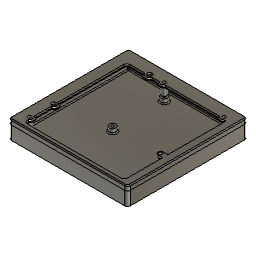
Lightroom-Macropad-Case (Autodesk Fusion 360 design; units mm, degrees)
Autodesk Fusion 360 part; units mm, degrees
(part 1 of 2)
sketch "BoardSVG" plane through (0, 0, 0) normal (0, 0, 1) x (1, 0, 0)
  ellipse E0 centre (-23.8658, -18.9665) end of major axis (-23.0959, -18.9665) minor radius 0.7699
  circle A0 centre (-23.8661, -18.9665) radius 0.5052
  ellipse E1 centre (-8.2045, -18.9665) end of major axis (-7.4346, -18.9665) minor radius 0.7699
  circle A1 centre (-8.2047, -18.9665) radius 0.5052
  ellipse E2 centre (-23.8658, -11.2672) end of major axis (-23.0959, -11.2672) minor radius 0.7699
  circle A2 centre (-23.8661, -11.2672) radius 0.5052
  ellipse E3 centre (-8.2045, -11.2672) end of major axis (-7.4346, -11.2672) minor radius 0.7699
  circle A3 centre (-8.2047, -11.2672) radius 0.5052
  ellipse E4 centre (-23.8658, -4.851) end of major axis (-23.0959, -4.851) minor radius 0.7699
  circle A4 centre (-23.8661, -4.851) radius 0.5052
  ellipse E5 centre (-8.2045, -4.851) end of major axis (-7.4346, -4.851) minor radius 0.7699
  circle A5 centre (-8.2047, -4.851) radius 0.5052
  ellipse E6 centre (-23.8658, 1.5651) end of major axis (-23.0959, 1.5651) minor radius 0.7699
  circle A6 centre (-23.8661, 1.5651) radius 0.5052
  ellipse E7 centre (-8.2045, 1.5651) end of major axis (-7.4346, 1.5651) minor radius 0.7699
  circle A7 centre (-8.2047, 1.5651) radius 0.5052
  ellipse E8 centre (66.4399, -35.8623) end of major axis (67.2482, -35.8623) minor radius 0.8083
  circle A8 centre (66.44, -35.8624) radius 0.4042
  ellipse E9 centre (74.7254, -35.8623) end of major axis (75.5338, -35.8623) minor radius 0.8083
  circle A9 centre (74.7254, -35.8624) radius 0.4042
  ellipse E10 centre (66.4399, -40.5676) end of major axis (67.2482, -40.5676) minor radius 0.8083
  circle A10 centre (66.44, -40.5676) radius 0.4042
  ellipse E11 centre (74.7254, -40.5676) end of major axis (75.5338, -40.5676) minor radius 0.8083
  circle A11 centre (74.7254, -40.5676) radius 0.4042
  ellipse E12 centre (66.4399, -45.2727) end of major axis (67.2482, -45.2727) minor radius 0.8083
  circle A12 centre (66.44, -45.2727) radius 0.4042
  ellipse E13 centre (74.7254, -45.2727) end of major axis (75.5338, -45.2727) minor radius 0.8083
  circle A13 centre (74.7254, -45.2727) radius 0.4042
  ellipse E14 centre (13.8275, 10.5477) end of major axis (14.6358, 10.5477) minor radius 0.8083
  circle A14 centre (13.8276, 10.5477) radius 0.4042
  ellipse E15 centre (22.113, 10.5477) end of major axis (22.9214, 10.5477) minor radius 0.8083
  circle A15 centre (22.113, 10.5477) radius 0.4042
  ellipse E16 centre (13.8275, 1.5651) end of major axis (14.6358, 1.5651) minor radius 0.8083
  circle A16 centre (13.8276, 1.5651) radius 0.4042
  ellipse E17 centre (22.113, 1.5651) end of major axis (22.9214, 1.5651) minor radius 0.8083
  circle A17 centre (22.113, 1.5651) radius 0.4042
  ellipse E18 centre (13.8275, -2.9262) end of major axis (14.6358, -2.9262) minor radius 0.8083
  circle A18 centre (13.8276, -2.9262) radius 0.4042
  ellipse E19 centre (22.113, -2.9262) end of major axis (22.9214, -2.9262) minor radius 0.8083
  circle A19 centre (22.113, -2.9262) radius 0.4042
  ellipse E20 centre (27.943, -45.2727) end of major axis (28.7513, -45.2727) minor radius 0.8083
  circle A20 centre (27.9431, -45.2727) radius 0.4042
  ellipse E21 centre (36.2286, -45.2727) end of major axis (37.0369, -45.2727) minor radius 0.8083
  circle A21 centre (36.2285, -45.2727) radius 0.4042
  ellipse E22 centre (27.943, -40.5674) end of major axis (28.7513, -40.5674) minor radius 0.8083
  circle A22 centre (27.9431, -40.5676) radius 0.4042
  ellipse E23 centre (36.2286, -40.5674) end of major axis (37.0369, -40.5674) minor radius 0.8083
  circle A23 centre (36.2285, -40.5676) radius 0.4042
  ellipse E24 centre (27.943, -31.1572) end of major axis (28.7513, -31.1572) minor radius 0.8083
  circle A24 centre (27.9431, -31.1572) radius 0.4042
  ellipse E25 centre (36.2286, -31.1572) end of major axis (37.0369, -31.1572) minor radius 0.8083
  circle A25 centre (36.2285, -31.1572) radius 0.4042
  ellipse E26 centre (27.943, -35.8623) end of major axis (28.7513, -35.8623) minor radius 0.8083
  circle A26 centre (27.9431, -35.8624) radius 0.4042
  ellipse E27 centre (36.2286, -35.8623) end of major axis (37.0369, -35.8623) minor radius 0.8083
  circle A27 centre (36.2285, -35.8624) radius 0.4042
  ellipse E28 centre (13.8275, -55.1107) end of major axis (14.6358, -55.1107) minor radius 0.8083
  circle A28 centre (13.8276, -55.1108) radius 0.4042
  ellipse E29 centre (22.113, -55.1107) end of major axis (22.9214, -55.1107) minor radius 0.8083
  circle A29 centre (22.113, -55.1108) radius 0.4042
  ellipse E30 centre (13.8275, -59.8161) end of major axis (14.6358, -59.8161) minor radius 0.8083
  circle A30 centre (13.8276, -59.816) radius 0.4042
  ellipse E31 centre (22.113, -59.8161) end of major axis (22.9214, -59.8161) minor radius 0.8083
  circle A31 centre (22.113, -59.816) radius 0.4042
  ellipse E32 centre (13.8275, -64.5212) end of major axis (14.6358, -64.5212) minor radius 0.8083
  circle A32 centre (13.8276, -64.5212) radius 0.4042
  ellipse E33 centre (22.113, -64.5212) end of major axis (22.9214, -64.5212) minor radius 0.8083
  circle A33 centre (22.113, -64.5212) radius 0.4042
  ellipse E34 centre (66.4399, -31.1572) end of major axis (67.2482, -31.1572) minor radius 0.8083
  circle A34 centre (66.44, -31.1572) radius 0.4042
  ellipse E35 centre (74.7254, -31.1572) end of major axis (75.5338, -31.1572) minor radius 0.8083
  circle A35 centre (74.7254, -31.1572) radius 0.4042
  ellipse E36 centre (13.8275, 6.0564) end of major axis (14.6358, 6.0564) minor radius 0.8083
  circle A36 centre (13.8276, 6.0564) radius 0.4042
  ellipse E37 centre (22.113, 6.0564) end of major axis (22.9214, 6.0564) minor radius 0.8083
  circle A37 centre (22.113, 6.0564) radius 0.4042
  ellipse E38 centre (13.8275, -50.4056) end of major axis (14.6358, -50.4056) minor radius 0.8083
  circle A38 centre (13.8276, -50.4056) radius 0.4042
  ellipse E39 centre (22.113, -50.4056) end of major axis (22.9214, -50.4056) minor radius 0.8083
  circle A39 centre (22.113, -50.4056) radius 0.4042
  ellipse E40 centre (-6.2799, -53.6137) end of major axis (-5.51, -53.6137) minor radius 0.7699
  circle A40 centre (-6.2797, -53.6137) radius 0.5052
  ellipse E41 centre (-21.941, -53.6137) end of major axis (-21.1711, -53.6137) minor radius 0.7699
  circle A41 centre (-21.9411, -53.6137) radius 0.5052
  ellipse E42 centre (17.9703, 16.1909) end of major axis (18.7402, 16.1909) minor radius 0.7699
  circle A42 centre (17.9703, 16.1909) radius 0.5052
  ellipse E43 centre (17.9703, 31.8522) end of major axis (18.7402, 31.8522) minor radius 0.7699
  circle A43 centre (17.9703, 31.8523) radius 0.5052
  ellipse E44 centre (-21.1682, -36.9317) end of major axis (-20.4609, -36.9317) minor radius 0.7073
  circle A44 centre (-21.1682, -36.9317) radius 0.4547
  ellipse E45 centre (-21.1682, -39.4982) end of major axis (-20.4609, -39.4982) minor radius 0.7073
  circle A45 centre (-21.1682, -39.4982) radius 0.4547
  ellipse E46 centre (3.2131, 40.7036) end of major axis (3.9204, 40.7036) minor radius 0.7073
  circle A46 centre (3.2131, 40.7036) radius 0.4547
  ellipse E47 centre (3.2131, 38.1372) end of major axis (3.9204, 38.1372) minor radius 0.7073
  circle A47 centre (3.2131, 38.1372) radius 0.4547
  ellipse E48 centre (17.9703, -15.1168) end of major axis (21.5067, -15.1168) minor radius 3.5365
  circle A48 centre (17.9703, -15.1168) radius 1.7965
  ellipse E49 centre (28.2361, 25.9465) end of major axis (29.4486, 25.9465) minor radius 1.2125
  circle A49 centre (28.2361, 25.9465) radius 0.8083
  ellipse E50 centre (34.6522, 28.5129) end of major axis (35.8647, 28.5129) minor radius 1.2125
  circle A50 centre (34.6522, 28.5129) radius 0.8083
  ellipse E51 centre (47.4845, 25.9465) end of major axis (48.697, 25.9465) minor radius 1.2125
  circle A51 centre (47.4845, 25.9465) radius 0.8083
  ellipse E52 centre (53.9007, 28.5129) end of major axis (55.1132, 28.5129) minor radius 1.2125
  circle A52 centre (53.9007, 28.5129) radius 0.8083
  ellipse E53 centre (-10.2608, -35.6485) end of major axis (-9.0483, -35.6485) minor radius 1.2125
  circle A53 centre (-10.2608, -35.6485) radius 0.8083
  ellipse E54 centre (-3.8446, -33.0821) end of major axis (-2.6321, -33.0821) minor radius 1.2125
  circle A54 centre (-3.8446, -33.0821) radius 0.8083
  ellipse E55 centre (8.9877, -35.6485) end of major axis (10.2002, -35.6485) minor radius 1.2125
  circle A55 centre (8.9877, -35.6485) radius 0.8083
  ellipse E56 centre (15.4038, -33.0821) end of major axis (16.6163, -33.0821) minor radius 1.2125
  circle A56 centre (15.4038, -33.0821) radius 0.8083
  ellipse E57 centre (66.733, -12.5504) end of major axis (67.9455, -12.5504) minor radius 1.2125
  circle A57 centre (66.733, -12.5504) radius 0.8083
  ellipse E58 centre (73.1491, -9.9839) end of major axis (74.3616, -9.9839) minor radius 1.2125
  circle A58 centre (73.1491, -9.9839) radius 0.8083
  ellipse E59 centre (66.733, 25.9465) end of major axis (67.9455, 25.9465) minor radius 1.2125
  circle A59 centre (66.733, 25.9465) radius 0.8083
  ellipse E60 centre (73.1491, 28.5129) end of major axis (74.3616, 28.5129) minor radius 1.2125
  circle A60 centre (73.1491, 28.5129) radius 0.8083
  ellipse E61 centre (47.4845, -54.8969) end of major axis (48.697, -54.8969) minor radius 1.2125
  circle A61 centre (47.4845, -54.8969) radius 0.8083
  ellipse E62 centre (53.9007, -52.3305) end of major axis (55.1132, -52.3305) minor radius 1.2125
  circle A62 centre (53.9007, -52.3305) radius 0.8083
  ellipse E63 centre (0.0051, -54.8969) end of major axis (1.2175, -54.8969) minor radius 1.2125
  circle A63 centre (0.0051, -54.8969) radius 0.8083
  ellipse E64 centre (6.4212, -52.3305) end of major axis (7.6337, -52.3305) minor radius 1.2125
  circle A64 centre (6.4212, -52.3305) radius 0.8083
  ellipse E65 centre (28.2361, -54.8969) end of major axis (29.4486, -54.8969) minor radius 1.2125
  circle A65 centre (28.2361, -54.8969) radius 0.8083
  ellipse E66 centre (34.6522, -52.3305) end of major axis (35.8647, -52.3305) minor radius 1.2125
  circle A66 centre (34.6522, -52.3305) radius 0.8083
  ellipse E67 centre (66.733, 6.6981) end of major axis (67.9455, 6.6981) minor radius 1.2125
  circle A67 centre (66.733, 6.6981) radius 0.8083
  ellipse E68 centre (73.1491, 9.2645) end of major axis (74.3616, 9.2645) minor radius 1.2125
  circle A68 centre (73.1491, 9.2645) radius 0.8083
  ellipse E69 centre (47.4845, -12.5504) end of major axis (48.697, -12.5504) minor radius 1.2125
  circle A69 centre (47.4845, -12.5504) radius 0.8083
  ellipse E70 centre (53.9007, -9.9839) end of major axis (55.1132, -9.9839) minor radius 1.2125
  circle A70 centre (53.9007, -9.9839) radius 0.8083
  ellipse E71 centre (28.2361, 6.6981) end of major axis (29.4486, 6.6981) minor radius 1.2125
  circle A71 centre (28.2361, 6.6981) radius 0.8083
  ellipse E72 centre (34.6522, 9.2645) end of major axis (35.8647, 9.2645) minor radius 1.2125
  circle A72 centre (34.6522, 9.2645) radius 0.8083
  ellipse E73 centre (66.733, -54.8969) end of major axis (67.9455, -54.8969) minor radius 1.2125
  circle A73 centre (66.733, -54.8969) radius 0.8083
  ellipse E74 centre (73.1491, -52.3305) end of major axis (74.3616, -52.3305) minor radius 1.2125
  circle A74 centre (73.1491, -52.3305) radius 0.8083
  ellipse E75 centre (28.2361, -12.5504) end of major axis (29.4486, -12.5504) minor radius 1.2125
  circle A75 centre (28.2361, -12.5504) radius 0.8083
  ellipse E76 centre (34.6522, -9.9839) end of major axis (35.8647, -9.9839) minor radius 1.2125
  circle A76 centre (34.6522, -9.9839) radius 0.8083
  ellipse E77 centre (47.4845, 6.6981) end of major axis (48.697, 6.6981) minor radius 1.2125
  circle A77 centre (47.4845, 6.6981) radius 0.8083
  ellipse E78 centre (53.9007, 9.2645) end of major axis (55.1132, 9.2645) minor radius 1.2125
  circle A78 centre (53.9007, 9.2645) radius 0.8083
  ellipse E79 centre (47.4845, -35.6485) end of major axis (48.697, -35.6485) minor radius 1.2125
  circle A79 centre (47.4845, -35.6485) radius 0.8083
  ellipse E80 centre (53.9007, -33.0821) end of major axis (55.1132, -33.0821) minor radius 1.2125
  circle A80 centre (53.9007, -33.0821) radius 0.8083
  ellipse E81 centre (17.9703, 38.7788) end of major axis (21.5067, 38.7788) minor radius 3.5365
  circle A81 centre (17.9703, 38.7788) radius 1.7965
  ellipse E82 centre (80.2069, 38.7788) end of major axis (83.7433, 38.7788) minor radius 3.5365
  circle A82 centre (80.2069, 38.7788) radius 1.7965
  ellipse E83 centre (-21.1682, -62.5963) end of major axis (-17.6318, -62.5963) minor radius 3.5365
  circle A83 centre (-21.1682, -62.5963) radius 1.7965
  ellipse E84 centre (80.2069, -27.3075) end of major axis (83.7433, -27.3075) minor radius 3.5365
  circle A84 centre (80.2069, -27.3075) radius 1.7965
  line L0 (-24.5046, 40.1903) -> (-22.9647, 40.1903)
  line L1 (-22.9647, 40.1903) -> (-22.9647, 38.6505)
  line L2 (-22.9647, 38.6505) -> (-24.5046, 38.6505)
  line L3 (-24.5046, 38.6505) -> (-24.5046, 40.1903)
  circle A85 centre (-23.7347, 39.4204) radius 0.462
  ellipse E85 centre (-23.7347, 36.8539) end of major axis (-22.9647, 36.8539) minor radius 0.7699
  circle A86 centre (-23.7347, 36.8539) radius 0.462
  ellipse E86 centre (-23.7347, 31.721) end of major axis (-22.9647, 31.721) minor radius 0.7699
  circle A87 centre (-23.7347, 31.721) radius 0.462
  ellipse E87 centre (-23.7347, 29.1546) end of major axis (-22.9647, 29.1546) minor radius 0.7699
  circle A88 centre (-23.7347, 29.1546) radius 0.462
  ellipse E88 centre (-23.7347, 26.5881) end of major axis (-22.9647, 26.5881) minor radius 0.7699
  circle A89 centre (-23.7347, 26.5881) radius 0.462
  ellipse E89 centre (-23.7347, 24.0216) end of major axis (-22.9647, 24.0216) minor radius 0.7699
  circle A90 centre (-23.7347, 24.0216) radius 0.462
  ellipse E90 centre (-23.7347, 21.4552) end of major axis (-22.9647, 21.4552) minor radius 0.7699
  circle A91 centre (-23.7347, 21.4552) radius 0.462
  ellipse E91 centre (-23.7347, 18.8887) end of major axis (-22.9647, 18.8887) minor radius 0.7699
  circle A92 centre (-23.7347, 18.8887) radius 0.462
  ellipse E92 centre (-23.7347, 16.3223) end of major axis (-22.9647, 16.3223) minor radius 0.7699
  circle A93 centre (-23.7347, 16.3223) radius 0.462
  ellipse E93 centre (-23.7347, 13.7558) end of major axis (-22.9647, 13.7558) minor radius 0.7699
  circle A94 centre (-23.7347, 13.7558) radius 0.462
  ellipse E94 centre (-23.7347, 11.1894) end of major axis (-22.9647, 11.1894) minor radius 0.7699
  circle A95 centre (-23.7347, 11.1894) radius 0.462
  ellipse E95 centre (-8.3359, 11.1894) end of major axis (-7.566, 11.1894) minor radius 0.7699
  circle A96 centre (-8.3359, 11.1894) radius 0.462
  ellipse E96 centre (-8.3359, 13.7558) end of major axis (-7.566, 13.7558) minor radius 0.7699
  circle A97 centre (-8.3359, 13.7558) radius 0.462
  ellipse E97 centre (-8.3359, 16.3223) end of major axis (-7.566, 16.3223) minor radius 0.7699
  circle A98 centre (-8.3359, 16.3223) radius 0.462
  ellipse E98 centre (-8.3359, 18.8887) end of major axis (-7.566, 18.8887) minor radius 0.7699
  circle A99 centre (-8.3359, 18.8887) radius 0.462
  ellipse E99 centre (-8.3359, 21.4552) end of major axis (-7.566, 21.4552) minor radius 0.7699
  circle A100 centre (-8.3359, 21.4552) radius 0.462
  ellipse E100 centre (-8.3359, 24.0216) end of major axis (-7.566, 24.0216) minor radius 0.7699
  circle A101 centre (-8.3359, 24.0216) radius 0.462
  ellipse E101 centre (-8.3359, 26.5881) end of major axis (-7.566, 26.5881) minor radius 0.7699
  circle A102 centre (-8.3359, 26.5881) radius 0.462
  ellipse E102 centre (-8.3359, 29.1546) end of major axis (-7.566, 29.1546) minor radius 0.7699
  circle A103 centre (-8.3359, 29.1546) radius 0.462
  ellipse E103 centre (-8.3359, 31.721) end of major axis (-7.566, 31.721) minor radius 0.7699
  circle A104 centre (-8.3359, 31.721) radius 0.462
  ellipse E104 centre (-8.3359, 34.2875) end of major axis (-7.566, 34.2875) minor radius 0.7699
  circle A105 centre (-8.3359, 34.2875) radius 0.462
  ellipse E105 centre (-8.3359, 36.8539) end of major axis (-7.566, 36.8539) minor radius 0.7699
  circle A106 centre (-8.3359, 36.8539) radius 0.462
  ellipse E106 centre (-8.3359, 39.4204) end of major axis (-7.566, 39.4204) minor radius 0.7699
  circle A107 centre (-8.3359, 39.4204) radius 0.462
  ellipse E107 centre (-23.7347, 34.2875) end of major axis (-22.9647, 34.2875) minor radius 0.7699
  circle A108 centre (-23.7347, 34.2875) radius 0.462
  ellipse E108 centre (-1.9198, -23.9578) end of major axis (-0.6568, -23.9578) minor radius 1.263
  circle A109 centre (-1.9198, -23.9578) radius 0.8083
  ellipse E109 centre (3.2131, -23.958) end of major axis (4.4761, -23.958) minor radius 1.263
  circle A110 centre (3.2131, -23.958) radius 0.8083
  ellipse E110 centre (8.346, -23.9578) end of major axis (9.6091, -23.9578) minor radius 1.263
  circle A111 centre (8.346, -23.9578) radius 0.8083
  ellipse E111 centre (0.6467, -6.2757) end of major axis (1.9097, -6.2757) minor radius 1.263
  circle A112 centre (0.6467, -6.2757) radius 0.8083
  ellipse E112 centre (5.7796, -6.2757) end of major axis (7.0426, -6.2757) minor radius 1.263
  circle A113 centre (5.7796, -6.2757) radius 0.8083
  arc A114 (-5.8806, -13.197) -> (-2.6474, -13.197) centre (-4.264, -13.2073) cw
  line L4 (-2.6474, -13.197) -> (-2.6474, -13.5002)
  arc A115 (-2.6474, -13.5002) -> (-5.8806, -13.5002) centre (-4.264, -13.4899) cw
  line L5 (-5.8806, -13.5002) -> (-5.8806, -13.197)
  arc A116 (-3.0514, -13.3991) -> (-5.4765, -13.3991) centre (-4.2639, -13.3991) cw
  line L6 (-5.4765, -13.3991) -> (-5.4765, -13.298)
  arc A117 (-5.4765, -13.298) -> (-3.0514, -13.298) centre (-4.2639, -13.298) cw
  line L7 (-3.0514, -13.298) -> (-3.0514, -13.3991)
  arc A118 (9.0736, -13.197) -> (12.3069, -13.197) centre (10.6903, -13.2073) cw
  line L8 (12.3069, -13.197) -> (12.3069, -13.5002)
  arc A119 (12.3069, -13.5002) -> (9.0736, -13.5002) centre (10.6903, -13.4899) cw
  line L9 (9.0736, -13.5002) -> (9.0736, -13.197)
  arc A120 (11.9027, -13.3991) -> (9.4776, -13.3991) centre (10.6902, -13.3991) cw
  line L10 (9.4776, -13.3991) -> (9.4776, -13.298)
  arc A121 (9.4776, -13.298) -> (11.9027, -13.298) centre (10.6902, -13.298) cw
  line L11 (11.9027, -13.298) -> (11.9027, -13.3991)
  ellipse E113 centre (-1.9198, 3.6316) end of major axis (-0.6568, 3.6316) minor radius 1.263
  circle A122 centre (-1.9198, 3.6316) radius 0.8083
  ellipse E114 centre (3.2131, 3.6314) end of major axis (4.4761, 3.6314) minor radius 1.263
  circle A123 centre (3.2131, 3.6314) radius 0.8083
  ellipse E115 centre (8.346, 3.6316) end of major axis (9.6091, 3.6316) minor radius 1.263
  circle A124 centre (8.346, 3.6316) radius 0.8083
  ellipse E116 centre (0.6467, 21.3138) end of major axis (1.9097, 21.3138) minor radius 1.263
  circle A125 centre (0.6467, 21.3138) radius 0.8083
  ellipse E117 centre (5.7796, 21.3138) end of major axis (7.0426, 21.3138) minor radius 1.263
  circle A126 centre (5.7796, 21.3138) radius 0.8083
  arc A127 (-5.8806, 14.3924) -> (-2.6474, 14.3924) centre (-4.264, 14.3821) cw
  line L12 (-2.6474, 14.3924) -> (-2.6474, 14.0893)
  arc A128 (-2.6474, 14.0893) -> (-5.8806, 14.0893) centre (-4.264, 14.0996) cw
  line L13 (-5.8806, 14.0893) -> (-5.8806, 14.3924)
  arc A129 (-3.0514, 14.1903) -> (-5.4765, 14.1903) centre (-4.2639, 14.1903) cw
  line L14 (-5.4765, 14.1903) -> (-5.4765, 14.2914)
  arc A130 (-5.4765, 14.2914) -> (-3.0514, 14.2914) centre (-4.2639, 14.2914) cw
  line L15 (-3.0514, 14.2914) -> (-3.0514, 14.1903)
  arc A131 (9.0736, 14.3924) -> (12.3069, 14.3924) centre (10.6903, 14.3821) cw
  line L16 (12.3069, 14.3924) -> (12.3069, 14.0893)
  arc A132 (12.3069, 14.0893) -> (9.0736, 14.0893) centre (10.6903, 14.0996) cw
  line L17 (9.0736, 14.0893) -> (9.0736, 14.3924)
  arc A133 (11.9027, 14.1903) -> (9.4776, 14.1903) centre (10.6902, 14.1903) cw
  line L18 (9.4776, 14.1903) -> (9.4776, 14.2914)
  arc A134 (9.4776, 14.2914) -> (11.9027, 14.2914) centre (10.6902, 14.2914) cw
  line L19 (11.9027, 14.2914) -> (11.9027, 14.1903)
  circle A135 centre (27.8396, 3.4733) radius 0.3082
  circle A136 centre (27.8396, 3.4733) radius 0.1541
  circle A137 centre (47.4576, -38.3589) radius 0.3082
  circle A138 centre (47.4576, -38.3589) radius 0.1541
  circle A139 centre (28.5045, 24.247) radius 0.3082
  circle A140 centre (28.5045, 24.247) radius 0.1541
  circle A141 centre (22.8011, 8.6693) radius 0.3082
  circle A142 centre (22.8011, 8.6693) radius 0.1541
  circle A143 centre (26.271, 4.7039) radius 0.3082
  circle A144 centre (26.271, 4.7039) radius 0.1541
  circle A145 centre (-7.4264, -0.6107) radius 0.3082
  circle A146 centre (-7.4264, -0.6107) radius 0.1541
  circle A147 centre (-15.7933, 7.1659) radius 0.3082
  circle A148 centre (-15.7933, 7.1659) radius 0.1541
  circle A149 centre (-3.6532, 5.7888) radius 0.3082
  circle A150 centre (-3.6532, 5.7888) radius 0.1541
  circle A151 centre (22.6764, -27.2341) radius 0.3082
  circle A152 centre (22.6764, -27.2341) radius 0.1541
  line L20 (-22.3231, 46.2215) -> (82.9017, 46.2215)
  line L21 (82.9017, -69.2691) -> (-22.3231, -69.2691)
  line L22 (-27.4561, -64.1362) -> (-27.4561, 41.0886)
  line L23 (88.0346, 41.0886) -> (88.0346, -64.1362)
  arc A153 (82.9017, 46.2215) -> (88.0346, 41.0886) centre (82.9017, 41.0886) cw
  arc A154 (88.0346, -64.1362) -> (82.9017, -69.2691) centre (82.9017, -64.1362) cw
  arc A155 (-22.3231, -69.2691) -> (-27.4561, -64.1362) centre (-22.3231, -64.1362) cw
  arc A156 (-27.4561, 41.0886) -> (-22.3231, 46.2215) centre (-22.3231, 41.0886) cw
  point P0 (-23.0959, -18.9665)
  point P1 (-23.3609, -18.9665)
  point P2 (-7.4346, -18.9665)
  point P3 (-7.6995, -18.9665)
  point P4 (-23.0959, -11.2672)
  point P5 (-23.3609, -11.2672)
  point P6 (-7.4346, -11.2672)
  point P7 (-7.6995, -11.2672)
  point P8 (-23.0959, -4.851)
  point P9 (-23.3609, -4.851)
  point P10 (-7.4346, -4.851)
  point P11 (-7.6995, -4.851)
  point P12 (-23.0959, 1.5651)
  point P13 (-23.3609, 1.5651)
  point P14 (-7.4346, 1.5651)
  point P15 (-7.6995, 1.5651)
  point P16 (67.2482, -35.8623)
  point P17 (66.8441, -35.8624)
  point P18 (75.5338, -35.8623)
  point P19 (75.1295, -35.8624)
  point P20 (67.2482, -40.5676)
  point P21 (66.8441, -40.5676)
  point P22 (75.5338, -40.5676)
  point P23 (75.1295, -40.5676)
  point P24 (67.2482, -45.2727)
  point P25 (66.8441, -45.2727)
  point P26 (75.5338, -45.2727)
  point P27 (75.1295, -45.2727)
  point P28 (14.6358, 10.5477)
  point P29 (14.2317, 10.5477)
  point P30 (22.9214, 10.5477)
  point P31 (22.5171, 10.5477)
  point P32 (14.6358, 1.5651)
  point P33 (14.2317, 1.5651)
  point P34 (22.9214, 1.5651)
  point P35 (22.5171, 1.5651)
  point P36 (14.6358, -2.9262)
  point P37 (14.2317, -2.9262)
  point P38 (22.9214, -2.9262)
  point P39 (22.5171, -2.9262)
  point P40 (28.7513, -45.2727)
  point P41 (28.3472, -45.2727)
  point P42 (37.0369, -45.2727)
  point P43 (36.6326, -45.2727)
  point P44 (28.7513, -40.5674)
  point P45 (28.3472, -40.5676)
  point P46 (37.0369, -40.5674)
  point P47 (36.6326, -40.5676)
  point P48 (28.7513, -31.1572)
  point P49 (28.3472, -31.1572)
  point P50 (37.0369, -31.1572)
  point P51 (36.6326, -31.1572)
  point P52 (28.7513, -35.8623)
  point P53 (28.3472, -35.8624)
  point P54 (37.0369, -35.8623)
  point P55 (36.6326, -35.8624)
  point P56 (14.6358, -55.1107)
  point P57 (14.2317, -55.1108)
  point P58 (22.9214, -55.1107)
  point P59 (22.5171, -55.1108)
  point P60 (14.6358, -59.8161)
  point P61 (14.2317, -59.816)
  point P62 (22.9214, -59.8161)
  point P63 (22.5171, -59.816)
  point P64 (14.6358, -64.5212)
  point P65 (14.2317, -64.5212)
  point P66 (22.9214, -64.5212)
  point P67 (22.5171, -64.5212)
  point P68 (67.2482, -31.1572)
  point P69 (66.8441, -31.1572)
  point P70 (75.5338, -31.1572)
  point P71 (75.1295, -31.1572)
  point P72 (14.6358, 6.0564)
  point P73 (14.2317, 6.0564)
  point P74 (22.9214, 6.0564)
  point P75 (22.5171, 6.0564)
  point P76 (14.6358, -50.4056)
  point P77 (14.2317, -50.4056)
  point P78 (22.9214, -50.4056)
  point P79 (22.5171, -50.4056)
  point P80 (-5.51, -53.6137)
  point P81 (-5.7745, -53.6137)
  point P82 (-21.1711, -53.6137)
  point P83 (-21.4359, -53.6137)
  point P84 (18.7402, 16.1909)
  point P85 (18.4755, 16.1909)
  point P86 (18.7402, 31.8522)
  point P87 (18.4755, 31.8523)
  point P88 (-20.4609, -36.9317)
  point P89 (-20.7135, -36.9317)
  point P90 (-20.4609, -39.4982)
  point P91 (-20.7135, -39.4982)
  point P92 (3.9204, 40.7036)
  point P93 (3.6678, 40.7036)
  point P94 (3.9204, 38.1372)
  point P95 (3.6678, 38.1372)
  point P96 (21.5067, -15.1168)
  point P97 (19.7668, -15.1168)
  point P98 (29.4486, 25.9465)
  point P99 (29.0444, 25.9465)
  point P100 (35.8647, 28.5129)
  point P101 (35.4606, 28.5129)
  point P102 (48.697, 25.9465)
  point P103 (48.2929, 25.9465)
  point P104 (55.1132, 28.5129)
  point P105 (54.709, 28.5129)
  point P106 (-9.0483, -35.6485)
  point P107 (-9.4524, -35.6485)
  point P108 (-2.6321, -33.0821)
  point P109 (-3.0363, -33.0821)
  point P110 (10.2002, -35.6485)
  point P111 (9.796, -35.6485)
  point P112 (16.6163, -33.0821)
  point P113 (16.2121, -33.0821)
  point P114 (67.9455, -12.5504)
  point P115 (67.5413, -12.5504)
  point P116 (74.3616, -9.9839)
  point P117 (73.9574, -9.9839)
  point P118 (67.9455, 25.9465)
  point P119 (67.5413, 25.9465)
  point P120 (74.3616, 28.5129)
  point P121 (73.9574, 28.5129)
  point P122 (48.697, -54.8969)
  point P123 (48.2929, -54.8969)
  point P124 (55.1132, -52.3305)
  point P125 (54.709, -52.3305)
  point P126 (1.2175, -54.8969)
  point P127 (0.8134, -54.8969)
  point P128 (7.6337, -52.3305)
  point P129 (7.2295, -52.3305)
  point P130 (29.4486, -54.8969)
  point P131 (29.0444, -54.8969)
  point P132 (35.8647, -52.3305)
  point P133 (35.4606, -52.3305)
  point P134 (67.9455, 6.6981)
  point P135 (67.5413, 6.6981)
  point P136 (74.3616, 9.2645)
  point P137 (73.9574, 9.2645)
  point P138 (48.697, -12.5504)
  point P139 (48.2929, -12.5504)
  point P140 (55.1132, -9.9839)
  point P141 (54.709, -9.9839)
  point P142 (29.4486, 6.6981)
  point P143 (29.0444, 6.6981)
  point P144 (35.8647, 9.2645)
  point P145 (35.4606, 9.2645)
  point P146 (67.9455, -54.8969)
  point P147 (67.5413, -54.8969)
  point P148 (74.3616, -52.3305)
  point P149 (73.9574, -52.3305)
  point P150 (29.4486, -12.5504)
  point P151 (29.0444, -12.5504)
  point P152 (35.8647, -9.9839)
  point P153 (35.4606, -9.9839)
  point P154 (48.697, 6.6981)
  point P155 (48.2929, 6.6981)
  point P156 (55.1132, 9.2645)
  point P157 (54.709, 9.2645)
  point P158 (48.697, -35.6485)
  point P159 (48.2929, -35.6485)
  point P160 (55.1132, -33.0821)
  point P161 (54.709, -33.0821)
  point P162 (21.5067, 38.7788)
  point P163 (19.7668, 38.7788)
  point P164 (83.7433, 38.7788)
  point P165 (82.0034, 38.7788)
  point P166 (-17.6318, -62.5963)
  point P167 (-19.3717, -62.5963)
  point P168 (83.7433, -27.3075)
  point P169 (82.0034, -27.3075)
  point P170 (-23.2727, 39.4204)
  point P171 (-22.9647, 36.8539)
  point P172 (-23.2727, 36.8539)
  point P173 (-22.9647, 31.721)
  point P174 (-23.2727, 31.721)
  point P175 (-22.9647, 29.1546)
  point P176 (-23.2727, 29.1546)
  point P177 (-22.9647, 26.5881)
  point P178 (-23.2727, 26.5881)
  point P179 (-22.9647, 24.0216)
  point P180 (-23.2727, 24.0216)
  point P181 (-22.9647, 21.4552)
  point P182 (-23.2727, 21.4552)
  point P183 (-22.9647, 18.8887)
  point P184 (-23.2727, 18.8887)
  point P185 (-22.9647, 16.3223)
  point P186 (-23.2727, 16.3223)
  point P187 (-22.9647, 13.7558)
  point P188 (-23.2727, 13.7558)
  point P189 (-22.9647, 11.1894)
  point P190 (-23.2727, 11.1894)
  point P191 (-7.566, 11.1894)
  point P192 (-7.874, 11.1894)
  point P193 (-7.566, 13.7558)
  point P194 (-7.874, 13.7558)
  point P195 (-7.566, 16.3223)
  point P196 (-7.874, 16.3223)
  point P197 (-7.566, 18.8887)
  point P198 (-7.874, 18.8887)
  point P199 (-7.566, 21.4552)
  point P200 (-7.874, 21.4552)
  point P201 (-7.566, 24.0216)
  point P202 (-7.874, 24.0216)
  point P203 (-7.566, 26.5881)
  point P204 (-7.874, 26.5881)
  point P205 (-7.566, 29.1546)
  point P206 (-7.874, 29.1546)
  point P207 (-7.566, 31.721)
  point P208 (-7.874, 31.721)
  point P209 (-7.566, 34.2875)
  point P210 (-7.874, 34.2875)
  point P211 (-7.566, 36.8539)
  point P212 (-7.874, 36.8539)
  point P213 (-7.566, 39.4204)
  point P214 (-7.874, 39.4204)
  point P215 (-22.9647, 34.2875)
  point P216 (-23.2727, 34.2875)
  point P217 (-0.6568, -23.9578)
  point P218 (-1.1115, -23.9578)
  point P219 (4.4761, -23.958)
  point P220 (4.0215, -23.958)
  point P221 (9.6091, -23.9578)
  point P222 (9.1544, -23.9578)
  point P223 (1.9097, -6.2757)
  point P224 (1.455, -6.2757)
  point P225 (7.0426, -6.2757)
  point P226 (6.5879, -6.2757)
  point P227 (-0.6568, 3.6316)
  point P228 (-1.1115, 3.6316)
  point P229 (4.4761, 3.6314)
  point P230 (4.0215, 3.6314)
  point P231 (9.6091, 3.6316)
  point P232 (9.1544, 3.6316)
  point P233 (1.9097, 21.3138)
  point P234 (1.455, 21.3138)
  point P235 (7.0426, 21.3138)
  point P236 (6.5879, 21.3138)
  point P237 (28.1478, 3.4733)
  point P238 (27.9937, 3.4733)
  point P239 (47.7658, -38.3589)
  point P240 (47.6117, -38.3589)
  point P241 (28.8127, 24.247)
  point P242 (28.6586, 24.247)
  point P243 (23.1093, 8.6693)
  point P244 (22.9552, 8.6693)
  point P245 (26.5791, 4.7039)
  point P246 (26.425, 4.7039)
  point P247 (-7.1182, -0.6107)
  point P248 (-7.2723, -0.6107)
  point P249 (-15.4851, 7.1659)
  point P250 (-15.6392, 7.1659)
  point P251 (-3.345, 5.7888)
  point P252 (-3.4991, 5.7888)
  point P253 (22.9846, -27.2341)
  point P254 (22.8305, -27.2341)
sketch "Base" plane through (0, 0, 0) normal (0, 0, 1) x (1, 0, 0)
  arc A0 (82.9017, -69.2691) -> (88.0346, -64.1362) centre (82.9017, -64.1362) ccw
  line L0 (82.9017, -69.2691) -> (-22.3231, -69.2691)
  arc A1 (-27.4561, -64.1362) -> (-22.3231, -69.2691) centre (-22.3231, -64.1362) ccw
  line L1 (-27.4561, -64.1362) -> (-27.4561, 41.0886)
  arc A2 (-22.3231, 46.2215) -> (-27.4561, 41.0886) centre (-22.3231, 41.0886) ccw
  line L2 (-22.3231, 46.2215) -> (82.9017, 46.2215)
  arc A3 (88.0346, 41.0886) -> (82.9017, 46.2215) centre (82.9017, 41.0886) ccw
  line L3 (88.0346, 41.0886) -> (88.0346, -64.1362)
  circle A4 centre (80.2069, 38.7788) radius 3.5365
  circle A5 centre (17.9703, 38.7788) radius 3.5365
  circle A6 centre (17.9703, -15.1168) radius 3.5365
  circle A7 centre (-21.1682, -62.5963) radius 3.5365
  circle A8 centre (80.2069, -27.3075) radius 3.5365
  circle A9 centre (17.9703, 38.7788) radius 1.5
  circle A10 centre (80.2069, 38.7788) radius 1.5
  circle A11 centre (-21.1682, -62.5963) radius 1.5
  circle A12 centre (17.9703, -15.1168) radius 1.5
  circle A13 centre (80.2069, -27.3075) radius 1.5
  line L4 (90.7573, 48.651) -> (90.7573, -72.4115)
  line L5 (90.7573, -72.4115) -> (-29.3052, -72.4115)
  line L6 (-29.3052, -72.4115) -> (-29.3052, 48.651)
  line L7 (-29.3052, 48.651) -> (90.7573, 48.651)
  line L8 (92.7573, 50.651) -> (92.7573, -74.4115)
  line L9 (92.7573, -74.4115) -> (-31.3052, -74.4115)
  line L10 (-31.3052, -74.4115) -> (-31.3052, 50.651)
  line L11 (-31.3052, 50.651) -> (92.7573, 50.651)
  point P0 (80.2069, -27.3075)
  point P1 (80.2069, -27.3075)
  dimension "d15" = 3
  dimension "d20" = 3
  constraint concentric A5 A9
  constraint concentric A4 A10
  constraint concentric A7 A11
  constraint concentric A6 A12
  constraint coincident P0 A8.centre
  measures "d15" diameter of A12
  measures "d20" diameter of A13
extrude "Extrude3" add sketch "Base" along normal blind 2 contours A0 L0 A1 L1 A2 L2 A3 L3 | A9 | A10 | A11 | A12 | A13 | L4 L5 L6 L7 makes body 1 at (19.3798, 38.2658, 1.3333) makes body 2 at (30.7828, -51.3146, 0) makes body 3 at (81.1994, 39.9035, 1.3333) makes body 4 at (19.4684, -15.1916, 1.3333) makes body 5 at (-19.7587, -63.1094, 1.3333) makes body 6 at (80.6131, -25.8636, 1.3333)
extrude "Extrude4" add sketch "Base" along normal blind 6.5 contours A4 | A5 | A6 | A7 | A8 bodies 1 2 3 4 5 6
extrude "Extrude7" add sketch "Base" along normal blind 14 contours L8 L9 L10 L11 bodies 1
sketch "USB Cutout" plane through (0, 48.651, 0) normal (0, -1, 0) x (1, 0, 0)
  line L0 (-29.3052, 2) -> (90.7573, 2)
  line L1 (90.7573, 2) -> (90.7573, 14)
  line L2 (90.7573, 14) -> (-29.3052, 14)
  line L3 (-29.3052, 14) -> (-29.3052, 2)
  line L4 (-6.8052, 10.75) -> (-23.8052, 10.75)
  line L5 (-23.8052, 10.75) -> (-23.8052, 17.25)
  line L6 (-23.8052, 17.25) -> (-6.8052, 17.25)
  line L7 (-6.8052, 17.25) -> (-6.8052, 10.75)
  line L8 (-6.8052, 10.75) -> (-23.8052, 17.25) construction
  line L9 (-23.8052, 10.75) -> (-6.8052, 17.25) construction
  point P0 (-15.3052, 14)
  dimension "d44" = 17
  dimension "d45" = 6.5
  constraint horizontal L4
  constraint perpendicular L4 L5
  constraint parallel L4 L6
  constraint parallel L5 L7
  constraint coincident L8 P0
  constraint coincident L9 P0
  measures "d44" distance of L5.end L6.end
  measures "d45" distance of L4.end L5.end
extrude "Extrude8" cut sketch "USB Cutout" against normal blind 6 contours L2 L4 L5 L7 bodies 1
sketch "Base Lip" plane through (0, 0, 14) normal (0, 0, 1) x (-1, 0, 0)
  line L0 (23.8052, -48.651) -> (23.8052, -50.651)
  line L1 (23.8052, -50.651) -> (31.3052, -50.651)
  line L2 (31.3052, -50.651) -> (31.3052, 74.4115)
  line L3 (31.3052, 74.4115) -> (-92.7573, 74.4115)
  line L4 (-92.7573, 74.4115) -> (-92.7573, -50.651)
  line L5 (-92.7573, -50.651) -> (6.8052, -50.651)
  line L6 (6.8052, -50.651) -> (6.8052, -48.651)
  line L7 (6.8052, -48.651) -> (-90.7573, -48.651)
  line L8 (-90.7573, -48.651) -> (-90.7573, 72.4115)
  line L9 (-90.7573, 72.4115) -> (29.3052, 72.4115)
  line L10 (29.3052, 72.4115) -> (29.3052, -48.651)
  line L11 (29.3052, -48.651) -> (23.8052, -48.651)
  line L12 (6.8052, -47.651) -> (-89.7573, -47.651)
  line L13 (-89.7573, -47.651) -> (-89.7573, 71.4115)
  line L14 (-89.7573, 71.4115) -> (28.3052, 71.4115)
  line L15 (28.3052, 71.4115) -> (28.3052, -47.651)
  line L16 (28.3052, -47.651) -> (23.8052, -47.651)
  line L17 (29.3052, -48.651) -> (23.8052, -48.651)
  line L18 (29.3052, 72.4115) -> (29.3052, -48.651)
  line L19 (6.8052, -48.651) -> (-90.7573, -48.651)
  line L20 (-90.7573, -48.651) -> (-90.7573, 72.4115)
  line L21 (-90.7573, 72.4115) -> (29.3052, 72.4115)
  line L22 (23.8052, -48.651) -> (23.8052, -47.651)
  line L23 (6.8052, -48.651) -> (6.8052, -47.651)
  dimension "d48" = 1
  constraint coincident L0.start L11.end
  constraint perpendicular L16 L22
  constraint coincident L6.end L7.start
  constraint perpendicular L12 L23
extrude "Extrude9" add sketch "Base Lip" along normal blind 3 separate body contours L7 L8 L9 L10 L11 L12 L13 L14 L15 L16 L17 L18 L19 L20 L21 L22 L23 makes body 7
extrude "Extrude10" add 1 faces at (-28.9719, -31.724, 14) along direction (0, 0, -1) blind 1 on bodies 7 bodies 7 1
chamfer "Chamfer1" distance 1 angle 45 5 edges at (-26.0552, 47.651, 13) (-28.3052, -11.8802, 13) (41.476, 47.651, 13) (89.7573, -11.8802, 13) (30.726, -71.4115, 13) on bodies 7
fillet "Fillet2" radius 3 4 edges at (92.7573, -74.4115, 7) (92.7573, 50.651, 7) (-31.3052, 50.651, 7) (-31.3052, -74.4115, 7) on bodies 7
fillet "Fillet3" radius 1 8 edges at (-29.3052, 48.651, 7.5) (-29.3052, -11.8802, 2) (30.726, 48.651, 2) (90.7573, 48.651, 7.5) (90.7573, -11.8802, 2) (90.7573, -72.4115, 7.5) (30.726, -72.4115, 2) (-29.3052, -72.4115, 7.5) on bodies 7
fillet "Fillet4" radius 1 8 edges at (90.7573, -72.4115, 15.5) (-29.3052, -72.4115, 15.5) (-29.3052, 48.651, 15.5) (90.7573, 48.651, 15.5) (-28.3052, -71.4115, 15.5) (-28.3052, 47.651, 15.5) (89.7573, 47.651, 15.5) (89.7573, -71.4115, 15.5) on bodies 7
fillet "Fillet5" radius 1 5 edges at (14.6731, -13.838, 2) (14.6731, 40.0576, 2) (-24.4654, -61.3175, 2) (76.9097, -26.0287, 2) (76.9097, 40.0576, 2) on bodies 1 7
chamfer "Chamfer2" distance 1 angle 45 3 edges at (-23.8052, 50.651, 12.375) (-15.3052, 50.651, 10.75) (-6.8052, 50.651, 12.375) on bodies 7
sketch "PCB Outline and Holes" plane through (0, 0, 6.5) normal (0, 0, 1) x (-1, 0, 0)
  arc A0 (-88.0346, -41.0886) -> (-82.9017, -46.2215) centre (-82.9017, -41.0886) ccw
  line L0 (-88.0346, -41.0886) -> (-88.0346, 64.1362)
  arc A1 (-82.9017, 69.2691) -> (-88.0346, 64.1362) centre (-82.9017, 64.1362) ccw
  line L1 (-82.9017, 69.2691) -> (22.3231, 69.2691)
  arc A2 (27.4561, 64.1362) -> (22.3231, 69.2691) centre (22.3231, 64.1362) ccw
  line L2 (27.4561, 64.1362) -> (27.4561, -41.0886)
  line L3 (22.3231, -46.2215) -> (-82.9017, -46.2215)
  arc A3 (22.3231, -46.2215) -> (27.4561, -41.0886) centre (22.3231, -41.0886) ccw
  circle A4 centre (21.1682, 62.5963) radius 1.75
  circle A5 centre (-80.2069, 27.3075) radius 1.75
  circle A6 centre (-17.9703, 15.1168) radius 1.75
  circle A7 centre (-17.9703, -38.7788) radius 1.75
  circle A8 centre (-80.2069, -38.7788) radius 1.75
  point P0 (-17.9703, -38.7788)
  point P1 (-80.2069, -38.7788)
  point P2 (-80.2069, 27.3075)
  point P3 (-17.9703, 15.1168)
  point P4 (21.1682, 62.5963)
  dimension "d66" = 3.5
  dimension "d67" = 3.5
  dimension "d68" = 3.5
  dimension "d69" = 3.5
  dimension "d70" = 3.5
  constraint coincident P4 A4.centre
  constraint coincident P2 A5.centre
  constraint coincident P3 A6.centre
  constraint coincident P0 A7.centre
  constraint coincident P1 A8.centre
  measures "d66" diameter of A4
  measures "d67" diameter of A5
  measures "d68" diameter of A6
  measures "d69" diameter of A7
  measures "d70" diameter of A8
extrude "Extrude11" add sketch "PCB Outline and Holes" along normal blind 1.78 separate body makes body 8
sketch "Lid Lip" plane through (0, 0, 14) normal (0, 0, 1) x (-1, 0, 0)
  line L0 (23.8052, -49.651) -> (24.8052, -50.651)
  line L1 (24.8052, -50.651) -> (28.3052, -50.651)
  arc A0 (28.3052, -50.651) -> (31.3052, -47.651) centre (28.3052, -47.651) ccw
  line L2 (31.3052, -47.651) -> (31.3052, 71.4115)
  arc A1 (31.3052, 71.4115) -> (28.3052, 74.4115) centre (28.3052, 71.4115) ccw
  line L3 (28.3052, 74.4115) -> (-89.7573, 74.4115)
  arc A2 (-89.7573, 74.4115) -> (-92.7573, 71.4115) centre (-89.7573, 71.4115) ccw
  line L4 (-92.7573, 71.4115) -> (-92.7573, -47.651)
  arc A3 (-92.7573, -47.651) -> (-89.7573, -50.651) centre (-89.7573, -47.651) ccw
  line L5 (-89.7573, -50.651) -> (5.8052, -50.651)
  line L6 (5.8052, -50.651) -> (6.8052, -49.651)
  line L7 (6.8052, -49.651) -> (6.8052, -48.651)
  line L8 (6.8052, -48.651) -> (-89.7573, -48.651)
  arc A4 (-90.7573, -47.651) -> (-89.7573, -48.651) centre (-89.7573, -47.651) ccw
  line L9 (-90.7573, -47.651) -> (-90.7573, 71.4115)
  arc A5 (-89.7573, 72.4115) -> (-90.7573, 71.4115) centre (-89.7573, 71.4115) ccw
  line L10 (-89.7573, 72.4115) -> (28.3052, 72.4115)
  arc A6 (29.3052, 71.4115) -> (28.3052, 72.4115) centre (28.3052, 71.4115) ccw
  line L11 (29.3052, 71.4115) -> (29.3052, -47.651)
  arc A7 (28.3052, -48.651) -> (29.3052, -47.651) centre (28.3052, -47.651) ccw
  line L12 (28.3052, -48.651) -> (23.8052, -48.651)
  line L13 (23.8052, -48.651) -> (23.8052, -49.651)
  line L14 (6.8052, -48.751) -> (-89.7573, -48.751)
  arc A8 (-90.8573, -47.651) -> (-89.7573, -48.751) centre (-89.7573, -47.651) ccw
  line L15 (-90.8573, -47.651) -> (-90.8573, 71.4115)
  arc A9 (-89.7573, 72.5115) -> (-90.8573, 71.4115) centre (-89.7573, 71.4115) ccw
  line L16 (-89.7573, 72.5115) -> (28.3052, 72.5115)
  arc A10 (29.4052, 71.4115) -> (28.3052, 72.5115) centre (28.3052, 71.4115) ccw
  line L17 (29.4052, 71.4115) -> (29.4052, -47.651)
  arc A11 (28.3052, -48.751) -> (29.4052, -47.651) centre (28.3052, -47.651) ccw
  line L18 (28.3052, -48.751) -> (23.8052, -48.751)
  dimension "d73" = 0.1
extrude "Extrude12" add sketch "Lid Lip" along normal blind 3 separate body contours L0 L1 A0 L2 A1 L3 A2 L4 A3 L5 L6 L7 L13 L14 A8 L15 A9 L16 A10 L17 A11 L18 makes body 9
sketch "Lid Face" plane through (0, 0, 17) normal (0, 0, 1) x (-1, 0, 0)
  line L0 (24.8052, -50.651) -> (28.3052, -50.651)
  arc A0 (28.3052, -50.651) -> (31.3052, -47.651) centre (28.3052, -47.651) ccw
  line L1 (31.3052, -47.651) -> (31.3052, 71.4115)
  arc A1 (31.3052, 71.4115) -> (28.3052, 74.4115) centre (28.3052, 71.4115) ccw
  line L2 (28.3052, 74.4115) -> (-89.7573, 74.4115)
  arc A2 (-89.7573, 74.4115) -> (-92.7573, 71.4115) centre (-89.7573, 71.4115) ccw
  line L3 (-92.7573, 71.4115) -> (-92.7573, -47.651)
  arc A3 (-92.7573, -47.651) -> (-89.7573, -50.651) centre (-89.7573, -47.651) ccw
  line L4 (-89.7573, -50.651) -> (5.8052, -50.651)
  line L5 (24.8052, -50.651) -> (5.8052, -50.651)
  circle A4 centre (-80.2069, 27.3075) radius 1.75
  circle A5 centre (-80.2069, -38.7788) radius 1.75
  circle A6 centre (-17.9703, -38.7788) radius 1.75
  circle A7 centre (21.1682, 62.5963) radius 1.75
  circle A8 centre (-17.9703, -38.7788) radius 2.75
  circle A9 centre (-80.2069, -38.7788) radius 2.75
  circle A10 centre (-80.2069, 27.3075) radius 2.75
  circle A11 centre (21.1682, 62.5963) radius 2.75
  line L6 (22.3231, -46.2215) -> (-82.9017, -46.2215)
  arc A12 (-88.0346, -41.0886) -> (-82.9017, -46.2215) centre (-82.9017, -41.0886) ccw
  line L7 (-88.0346, -41.0886) -> (-88.0346, 64.1362)
  arc A13 (-82.9017, 69.2691) -> (-88.0346, 64.1362) centre (-82.9017, 64.1362) ccw
  line L8 (-82.9017, 69.2691) -> (22.3231, 69.2691)
  arc A14 (27.4561, 64.1362) -> (22.3231, 69.2691) centre (22.3231, 64.1362) ccw
  arc A15 (22.3231, -46.2215) -> (27.4561, -41.0886) centre (22.3231, -41.0886) ccw
  line L9 (27.4561, 64.1362) -> (27.4561, -41.0886)
  line L10 (-88.0346, 24.5575) -> (-80.2069, 24.5575)
  circle A16 centre (-80.2069, 27.3075) radius 4.5365
  line L11 (-80.2069, 30.0575) -> (-84.1207, 30.0575)
  line L12 (-80.2069, -38.7788) -> (-80.2069, -41.5288)
  line L13 (-80.2069, -38.7788) -> (-80.2069, -36.0288)
  line L14 (-80.2069, -36.0288) -> (-88.0346, -36.0288)
  line L15 (-80.2069, -36.0288) -> (-77.4569, -36.0288)
  line L16 (-80.2069, -41.5288) -> (-88.0157, -41.5288)
  line L17 (-80.2069, -41.5288) -> (-77.4569, -41.5288)
  line L18 (-77.4569, -38.7788) -> (-77.4569, -41.5288)
  line L19 (-77.4569, -38.7788) -> (-77.4569, -36.0288)
  circle A17 centre (-80.2069, -38.7788) radius 4.5365
  circle A18 centre (-17.9703, -38.7788) radius 4.5365
  line L20 (18.4182, 62.5963) -> (18.4182, 69.2691)
  line L21 (28.3052, -46.651) -> (28.3052, 70.4115)
  line L22 (21.1682, 59.8463) -> (27.4561, 59.8463)
  arc A19 (18.4182, 66.2042) -> (24.7761, 59.8463) centre (21.1682, 62.5963) ccw
  line L23 (-20.7203, -38.7788) -> (-20.7203, -46.2215)
  line L24 (-15.2203, -38.7788) -> (-15.2203, -46.2215)
  line L25 (28.3052, -47.651) -> (-89.7573, -47.651)
  line L26 (18.4182, 69.2691) -> (18.4182, 62.5963)
  line L27 (-77.4569, -36.0288) -> (18.4182, -36.0288)
  line L28 (18.4182, 58.9884) -> (18.4182, -36.0288)
  line L29 (-84.1207, -36.0288) -> (-84.1207, 24.5575)
  line L30 (-84.1207, 30.0575) -> (-84.1207, 33)
  line L31 (-84.1207, 33) -> (-84.1207, 46.0807)
  line L32 (-84.1207, 46.0807) -> (-84.1207, 69.1222)
  dimension "d78" = 1
  dimension "d79" = 1
  dimension "d80" = 1
  dimension "d82" = 1
  constraint coincident L0.start L5.start
  constraint coincident L4.end L5.end
  constraint coincident L7 L10.start
  constraint coincident A10 L11.start
  constraint perpendicular L7 L11
  constraint coincident A5.centre A9.centre
  constraint coincident A9 L12.end
  constraint vertical L12
  constraint coincident A9 L13.end
  constraint parallel L12 L13
  constraint coincident A9 L18.start
  constraint coincident L7 L14.end
  constraint tangent A9 L14
  constraint tangent A9 L15
  constraint coincident A12 L16.end
  constraint tangent A9 L16
  constraint tangent A9 L17
  constraint tangent A9 L18
  constraint tangent A9 L19
  constraint concentric A5 A17
  constraint concentric A6 A18
  constraint concentric A7 A19
  constraint coincident A11 L20.start
  constraint tangent A11 L20
  constraint perpendicular L8 L20
  constraint coincident A11 L22.start
  constraint tangent A11 L22
  constraint perpendicular L9 L22
  constraint coincident L9 L22.end
  constraint coincident L8 L20.end
  constraint coincident L22 A19.end
  constraint coincident L20 A19.start
  constraint coincident A8 L23.start
  constraint coincident L6 L23.end
  constraint tangent A8 L23
  constraint perpendicular L6 L23
  constraint coincident A8 L24.start
  constraint coincident L6 L24.end
  constraint tangent A8 L24
  constraint perpendicular L6 L24
  constraint perpendicular L6 L26
  constraint coincident A19 L28.start
  constraint collinear L26 L28
  constraint perpendicular L27 L28
  constraint midpoint L14 L29.start
  constraint perpendicular L11 L29
  constraint collinear L29 L30
  constraint coincident L10 L29.end
  constraint parallel L30 L31
  constraint coincident A13 L32.end
  constraint parallel L31 L32
  constraint coincident A10 L10.end
extrude "Extrude13" add sketch "Lid Face" along normal blind 2 contours L0 A0 L1 A1 L2 A2 L3 A3 L4 L5 | A4 | A5 L12 L13 | A5 A9 L12 L13 | A5 L12 L13 | A5 A9 L12 L13 | A9 L15 L19 | A9 L14 L16 A17 | L14 L15 A17 L27 | L16 L17 L18 L19 A17 L27 | A9 L17 L18 | A12 L7 L14 L16 A17 | A13 L8 L10 A16 L11 L14 A17 A18 L20 A19 L26 L27 L28 L29 L30 L31 L32 | L6 A12 L16 A17 A18 L23 L27 | L7 L10 L14 L29 | L7 A13 L10 A16 L11 L30 L31 L32 | A8 A18 L23 L27 | A18 L27 | A10 L10 A16 L11 | A10 L10 A16 L11 | L6 A15 L9 A18 L22 A19 L24 L27 L28 | A8 A18 L24 L27 | A8 A18 L23 L24 | L6 A18 L23 L24 | A8 | A10 | A11 L20 L22 A19 L26 | A11 L8 A14 L9 L20 L22 L26 | A11 | A6 | A7 bodies 9
extrude "Extrude14" add sketch "Lid Face" against normal blind 8.72 separate body contours A5 A9 L12 L13 | A5 A9 L12 L13 | A8 | A10 | A11 makes body 10 at (82.5534, 37.3448, 14.0933) makes body 11 at (15.2339, 38.505, 14.0933) makes body 12 at (82.5534, -28.7415, 14.0933) makes body 13 at (-23.9046, -62.3225, 11.1867)
combine "Combine1" operation add target body 9 tool bodies 10 12 13 11
sketch "Sketch12" plane through (0, 0, 19) normal (0, 0, 1) x (-1, 0, 0)
  circle A0 centre (-17.9703, -38.7788) radius 1.75
  circle A1 centre (-80.2069, -38.7788) radius 1.75
  circle A2 centre (-80.2069, 27.3075) radius 1.75
  circle A3 centre (21.1682, 62.5963) radius 1.75
  arc A4 (28.3052, -50.651) -> (31.3052, -47.651) centre (28.3052, -47.651) ccw
  line L0 (31.3052, -47.651) -> (31.3052, 71.4115)
  arc A5 (31.3052, 71.4115) -> (28.3052, 74.4115) centre (28.3052, 71.4115) ccw
  line L1 (28.3052, 74.4115) -> (-89.7573, 74.4115)
  arc A6 (-89.7573, 74.4115) -> (-92.7573, 71.4115) centre (-89.7573, 71.4115) ccw
  line L2 (-92.7573, 71.4115) -> (-92.7573, -47.651)
  arc A7 (-92.7573, -47.651) -> (-89.7573, -50.651) centre (-89.7573, -47.651) ccw
  line L3 (-89.7573, -50.651) -> (28.3052, -50.651)
  circle A8 centre (-3.2131, -38.4204) radius 2.5
  circle A9 centre (20.1682, 38.215) radius 2.5
  circle A10 centre (-3.2131, -38.4204) radius 5.1781
  circle A11 centre (20.1682, 38.215) radius 4.5365
  line L4 (18.4197, 34.029) -> (18.462, 42.4183)
  line L5 (1.3833, -36.0359) -> (-7.8936, -36.2056)
  point P0 (-3.2131, -38.1372)
  point P1 (-3.2131, -40.7036)
  point P2 (21.1682, 39.4982)
  point P3 (21.1682, 36.9317)
  dimension "d95" = 5
  dimension "d96" = 5
  constraint concentric A8 A10
  constraint concentric A9 A11
  constraint coincident A11 L4.start
  constraint coincident A11 L4.end
  constraint coincident A10 L5.start
  constraint coincident A10 L5.end
  measures "d95" diameter of A8
  measures "d96" diameter of A9
extrude "Extrude17" cut sketch "Sketch12" against normal blind 22 contours A0 | A1 | A2 | A3 bodies 9
extrude "Extrude22" cut sketch "Lid Face" along normal blind 2 contours A13 L8 L10 A16 L11 L14 A17 A18 L20 A19 L26 L27 L28 L29 L30 L31 L32 | A10 L10 A16 L11 picked at (-80.1084, 31.2388) bodies 9
extrude "Extrude23" cut sketch "Sketch12" against normal blind 2 contours A8 L5 | A8 L5 | A9 L4 | A9 L4 bodies 9
extrude "Extrude24" add sketch "Sketch12" against normal blind 2 contours A8 A10 L5 | A9 A11 L4 picked at (-3.2913, -34.1452) picked at (16.3279, 37.9509) bodies 9
fillet "Fillet8" radius 1 4 edges at (82.9569, -27.3075, 17) (82.7708, 39.7732, 17) (20.5342, 39.7732, 17) (-18.6043, -61.6019, 17) on bodies 9
fillet "Fillet9" radius 3 3 edges at (-18.4182, 36.0288, 18) (-18.4182, -69.2691, 18) (84.1207, -69.1222, 18) on bodies 9
chamfer "Chamfer6" distance 1 angle 45 25 edges at (30.726, 50.651, 19) (-30.4265, 49.7724, 19) (-31.3052, -11.8802, 19) (-30.4265, -73.5328, 19) (30.726, -74.4115, 19) (91.8786, -73.5328, 19) (92.7573, -11.8802, 19) (91.8786, 49.7724, 19) (-18.4182, -50.6944, 19) (-16.6318, -62.5963, 19) (32.8512, -69.2691, 19) (-17.5395, -68.3904, 19) (-18.4182, -66.2367, 19) (84.1207, -48.1633, 19) (83.242, -68.3904, 19) (-15.6318, -38.215, 19) (-18.4182, -0.5004, 19) (-17.5395, 35.1501, 19) (-8.3989, 36.0288, 19) (3.2131, 33.2423, 19) (11.0841, 36.0288, 19) (17.9703, 34.2423, 19) (49.0886, 36.0288, 19) (80.2069, 34.2423, 19) (84.1207, 5.7356, 19) on bodies 9
hidden bodies 8
equation "InnerDepth = 12 mm"
equation "MaterialThickness = 2 mm"
equation "PostHeight = 4.5 mm"
equation "PostDiameter = 7.5 mm"
equation "PostInnerDiameter = 3 mm"
equation "OuterBuffer = 2 mm"
equation "d15 = PostInnerDiameter"
equation "d20 = PostInnerDiameter"
equation "d21 = MaterialThickness"
equation "d23 = MaterialThickness + PostHeight"
equation "USB_Height = 6.5 mm"
equation "USB_Width = 17 mm"
equation "USB_Left_Margin = 14 mm" comment "To center"
equation "USB_Bottom_Margin = 12 mm" comment "To center"
equation "d39 = -MaterialThickness"
equation "d40 = MaterialThickness + InnerDepth"
equation "d44 = USB_Width"
equation "d45 = USB_Height"